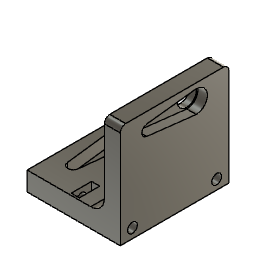
Wrist 1 Side 2 Rev4 (Autodesk Fusion 360 design; units mm, degrees)
Autodesk Fusion 360 part; units mm, degrees
note: some values were not read from the file. Chosen so that the rebuilt part matches the saved one: which face or edge a step refers to. Set by a fixed rule: which sketch regions a step uses.
sketch "Sketch9" plane through (0, 0, 0) normal (0, 0, 1) x (1, 0, 0)
  line L0 (0, 0) -> (27.32, 0)
  line L1 (27.32, 0) -> (27.32, 40)
  line L2 (27.32, 40) -> (0, 40)
  line L3 (0, 40) -> (0, 0)
  line L4 (27.32, 0) -> (21.42, 0)
  line L5 (21.42, 0) -> (21.42, 40)
  line L6 (21.42, 40) -> (27.32, 40)
  line L7 (27.32, 40) -> (27.32, 0)
  circle A0 centre (0, 28) radius 3.55
  circle A1 centre (0, 28) radius 4.1
  line L8 (0, 28) -> (4.1, 28)
  line L9 (0, 28) -> (-4.1, 28)
  line L10 (4.1, 28) -> (1.9867, 9.7387)
  circle A2 centre (0, 9.9686) radius 2
  line L11 (-4.1, 28) -> (-1.9867, 9.7387)
  line L12 (0, 40) -> (-7, 40)
  line L13 (-7, 40) -> (-7, 0)
  line L14 (-7, 0) -> (0, 0)
  line L15 (0, 0) -> (0, 40)
  dimension "d74" = 40
  dimension "d75" = 27.32
  dimension "d76" = 5.9
  dimension "d77" = 7.1
  dimension "d78" = 12
  dimension "d79" = 8.2
  dimension "d81" = 4
  dimension "d124" = 7
  constraint horizontal L0
  constraint vertical L1
  constraint horizontal L2
  constraint vertical L3
  constraint coincident L0.start L3.end
  constraint horizontal L4
  constraint vertical L5
  constraint horizontal L6
  constraint vertical L7
  constraint coincident L3 A0.centre
  constraint concentric A0 A1
  constraint coincident A0.centre A1.centre
  constraint coincident A1 L8.end
  constraint perpendicular L3 L8
  constraint coincident A1 L9.end
  constraint parallel L8 L9
  constraint coincident L3 A2.centre
  constraint coincident L10.end A2
  constraint tangent L10 A2
  constraint coincident A2 L11.end
  constraint tangent A2 L11
  constraint horizontal L12
  constraint vertical L13
  constraint horizontal L14
  constraint vertical L15
  measures "d74" distance of L0.start L2.end
  measures "d75" distance of L0.start L0.end
  measures "d76" distance of L0.end L4.end
  measures "d77" diameter of A0
  measures "d78" distance of L2 A0.centre
  measures "d79" diameter of A1
  measures "d81" diameter of A2
  measures "d124" distance of L13.end L0.start
extrude "Extrude14" add sketch "Sketch9" along normal blind 7 contours L0 L2 L3 L5 A1 L10 A2 L15 | L3 A1 A2 L11 L12 L13 L14 L15 | L0 L1 L2 L4 L5 L6 L7
extrude "Extrude15" add sketch "Sketch9" along normal blind 2.5 contours L3 A2 L15 | L3 A2 L15 | L3 A1 A2 L11 L15 | L3 A1 L10 A2 L15 | L3 A0 A1 L9 L11 L15 | L3 A0 A1 L8 L10 L15 | L3 A0 A1 L8 L15 | L3 A0 A1 L9 L15
extrude "Extrude16" add sketch "Sketch9" along normal blind 38 contours L0 L1 L2 L4 L5 L6 L7
fillet "Fillet6" radius 5 1 edges at (21.42, 20, 7)
sketch "Sketch11" plane through (27.32, 0, 0) normal (1, 0, 0) x (0, 1, 0)
  line L0 (0, 0) -> (40, 0)
  line L1 (40, 0) -> (40, 38)
  line L2 (40, 38) -> (0, 38)
  line L3 (0, 38) -> (0, 0)
  line L4 (28, 32) -> (28, 27.9)
  line L5 (28, 36.1) -> (9.7387, 33.9867)
  circle A0 centre (28, 32) radius 3.55
  line L6 (28, 27.9) -> (9.7387, 30.0133)
  line L7 (28, 32) -> (28, 36.1)
  circle A1 centre (28, 32) radius 4.1
  circle A2 centre (9.9686, 32) radius 2
  circle A3 centre (28, 32) radius 3.1
  dimension "d98" = 7.1
  dimension "d99" = 8.2
  dimension "d100" = 4
  dimension "d105" = 6.2
  constraint concentric A0 A1
  constraint coincident L4.start A0.centre
  constraint coincident L4.end A1
  constraint coincident L5.start A1
  constraint parallel L4 L7
  constraint coincident L6.end A2
  constraint tangent L6 A2
  constraint coincident L5.end A2
  constraint tangent L5 A2
  measures "d98" diameter of A0
  measures "d99" diameter of A1
  measures "d100" diameter of A2
  measures "d105" diameter of A3
extrude "Extrude18" cut sketch "Sketch11" against normal up to surface (5.9 mm away) contours L4 L7 A3 | L4 L7 A3 | L4 A0 L7 A3 | L4 A0 L7 A3
extrude "Extrude19" cut sketch "Sketch11" against normal blind 3.5 contours L4 A0 L7 A1 | L4 L5 A0 L6 L7 A1 | L5 L6 A1 A2 | A2
fillet "Fillet9" radius 2 1 edges at (24.37, 0, 38)
fillet "Fillet10" radius 2 1 edges at (24.37, 40, 38)
sketch "Sketch13" plane through (-7, 0, 0) normal (-1, 0, 0) x (0, -1, 0)
  line L0 (-40, 0) -> (0, 0)
  line L1 (0, 0) -> (0, 7)
  line L2 (0, 7) -> (-40, 7)
  line L3 (-40, 7) -> (-40, 0)
  line L4 (0, 3.5) -> (-4.5, 3.5)
  line L5 (-40, 3.5) -> (-35.5, 3.5)
  circle A0 centre (-35.5, 3.5) radius 1.8
  circle A1 centre (-4.5, 3.5) radius 1.8
  dimension "d125" = 4.5
  dimension "d126" = 4.5
  dimension "d127" = 3.6
  dimension "d128" = 3.6
  constraint midpoint L1 L4.start
  constraint perpendicular L1 L4
  constraint midpoint L3 L5.start
  constraint perpendicular L3 L5
  constraint coincident L5.end A0.centre
  constraint coincident L4.end A1.centre
  measures "d125" distance of L4.start L4.end
  measures "d126" distance of L5.start L5.end
  measures "d127" diameter of A0
  measures "d128" diameter of A1
extrude "Extrude22" cut sketch "Sketch13" against normal up to surface (34.32 mm away) contours A0 | A1
sketch "Sketch14" plane through (0, 0, 7) normal (0, 0, 1) x (-1, 0, 0)
  line L0 (-16.42, 0) -> (-16.42, -40)
  line L1 (-16.42, -40) -> (7, -40)
  line L2 (7, -40) -> (7, 0)
  line L3 (7, 0) -> (-16.42, 0)
  arc A0 (-3.9916, -27.0636) -> (3.9916, -27.0636) centre (0, -28) ccw
  line L4 (-3.9916, -27.0636) -> (-1.9867, -9.7387)
  arc A1 (1.9867, -9.7387) -> (-1.9867, -9.7387) centre (0, -9.9686) ccw
  line L5 (1.9867, -9.7387) -> (3.9916, -27.0636)
  line L6 (-10.0028, -40) -> (-10.0028, -35.5)
  line L7 (-10, 0) -> (-10, -4.5)
  line L8 (-8.5028, -39.25) -> (-11.5028, -39.25)
  line L9 (-11.5028, -39.25) -> (-11.5028, -31.75)
  line L10 (-11.5028, -31.75) -> (-8.5028, -31.75)
  line L11 (-8.5028, -31.75) -> (-8.5028, -39.25)
  line L12 (-8.5028, -39.25) -> (-11.5028, -31.75) construction
  line L13 (-11.5028, -39.25) -> (-8.5028, -31.75) construction
  line L14 (-11.5, -8.25) -> (-8.5, -8.25)
  line L15 (-8.5, -8.25) -> (-8.5, -0.75)
  line L16 (-8.5, -0.75) -> (-11.5, -0.75)
  line L17 (-11.5, -0.75) -> (-11.5, -8.25)
  line L18 (-11.5, -8.25) -> (-8.5, -0.75) construction
  line L19 (-8.5, -8.25) -> (-11.5, -0.75) construction
  point P0 (-10.0028, -35.5)
  point P1 (-10, -4.5)
  dimension "d131" = 4.5
  dimension "d132" = 4.5
  dimension "d133" = 3
  dimension "d134" = 7.5
  dimension "d135" = 3
  dimension "d136" = 7.5
  constraint coincident L1 L6.start
  constraint perpendicular L1 L6
  constraint coincident L3 L7.start
  constraint perpendicular L3 L7
  constraint horizontal L8
  constraint perpendicular L8 L9
  constraint parallel L8 L10
  constraint parallel L9 L11
  constraint coincident L12 P0
  constraint coincident L13 P0
  constraint coincident P0 L6.end
  constraint horizontal L14
  constraint perpendicular L14 L15
  constraint parallel L14 L16
  constraint parallel L15 L17
  constraint coincident L18 P1
  constraint coincident L19 P1
  constraint coincident P1 L7.end
  measures "d131" distance of L6.start P0
  measures "d132" distance of L7.start P1
  measures "d133" distance of L9.end L10.end
  measures "d134" distance of L8.start L10.end
  measures "d135" distance of L15.end L16.end
  measures "d136" distance of L14.end L15.end
extrude "Extrude23" cut sketch "Sketch14" against normal up to surface (7 mm away) contours L8 L9 L10 L11 | L14 L15 L16 L17
